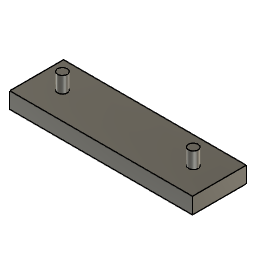
wire_linear_bus (Autodesk Fusion 360 design; units mm, degrees)
part number: 2025-07-06-17-30-28-126
Autodesk Fusion 360 part; units mm, degrees
note: some values were not read from the file. Set by a fixed rule: which sketch regions a step uses.
sketch "Schizzo1" plane through (0, 0, 0) normal (0, 0, 1) x (1, 0, 0)
  line L0 (0, 0) -> (-56.8, 0)
  line L1 (-56.8, 0) -> (-56.8, 16.7)
  line L2 (-56.8, 16.7) -> (0, 16.7)
  line L3 (0, 16.7) -> (0, 0)
  line L4 (0, 0) -> (0, 8.35)
  line L5 (0, 8.35) -> (-56.8, 8.35)
  line L6 (-56.8, 8.35) -> (-48.7, 8.35)
  line L7 (0, 8.35) -> (-8.1, 8.35)
  circle A0 centre (-48.7, 8.35) radius 1.5
  circle A1 centre (-8.1, 8.35) radius 1.5
  dimension "d1" = 56.8
  dimension "d2" = 16.7
  dimension "d3" = 8.1
  dimension "d4" = 8.1
  dimension "d5" = 3
  dimension "d6" = 3
  constraint horizontal L0
  constraint vertical L1
  constraint horizontal L2
  constraint vertical L3
  constraint coincident L0.start L3.end
  constraint midpoint L3 L4.end
  constraint midpoint L1 L5.end
  constraint perpendicular L1 L6
  constraint perpendicular L4 L7
  constraint coincident L6.end A0.centre
  constraint coincident L7.end A1.centre
  measures "d1" distance of L0.start L0.end
  measures "d2" distance of L0.start L2.end
  measures "d3" distance of L5.end L6.end
  measures "d4" distance of L4.end L7.end
  measures "d5" diameter of A0
  measures "d6" diameter of A1
extrude "Estrusione1" add sketch "Schizzo1" along normal blind 10 contours L5 L7 A1 | L5 L7 A1 | L5 L6 A0 | L5 L6 A0 makes body 1 at (-48.4395, 6.8728, 6.6667) makes body 2 at (-6.6075, 8.4994, 6.6667)
sketch "Schizzo2" plane through (0, 0, 0) normal (0, 0, 1) x (1, 0, 0)
  line L0 (0, 0) -> (-56.7, 0)
  line L1 (-56.7, 0) -> (-56.7, 16.7)
  line L2 (-56.7, 16.7) -> (0, 16.7)
  line L3 (0, 16.7) -> (0, 0)
  dimension "d9" = 56.7
  dimension "d10" = 16.7
  constraint horizontal L0
  constraint vertical L1
  constraint horizontal L2
  constraint vertical L3
  constraint coincident L0.start L3.end
  measures "d9" distance of L0.start L0.end
  measures "d10" distance of L0.start L2.end
extrude "Estrusione2" add sketch "Schizzo2" along normal blind 5 bodies 1 2
